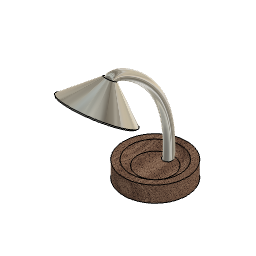
lamp-f3d (Autodesk Fusion 360 design; units mm, degrees)
Autodesk Fusion 360 part; units mm, degrees
sketch "Sketch1" plane through (0, 0, 0) normal (0, 0, 1) x (1, 0, 0)
  circle A0 centre (0, 0) radius 60
  circle A1 centre (0, 0) radius 47.5
  line L0 (-47.5, 0) -> (47.5, 0) construction
  line L1 (0, 0) -> (0, 47.5) construction
  circle A2 centre (0, 23.75) radius 8.5
  dimension "d1" = 120
  dimension "d2" = -12.5
  dimension "d3" = 17
  constraint coincident A0.centre A1.centre
  constraint coincident A1 L0.start
  constraint coincident A1 L0.end
  constraint horizontal L0
  constraint coincident A1 L1.end
  constraint perpendicular L0 L1
  constraint midpoint L1 A2.centre
  measures "d1" diameter of A0
  measures "d3" diameter of A2
extrude "Extrude1" add sketch "Sketch1" along normal blind 30 contours A0 makes body 1
extrude "Extrude2" add sketch "Sketch1" along normal blind 20 contours A1 bodies 1
fillet "Fillet1" radius 15 1 edges at (-44.2855, 17.1767, 20) on bodies 1
sketch "Sketch2" plane through (0, 0, 0) normal (1, 0, 0) x (0, 1, 0)
  spline S0 degree 5 poles (23.75, 0) (24.3992, 5.1936) (25.4927, 15.4647) (26.5181, 30.5229) (26.6466, 49.8986) (24.696, 72.9054) (20.5876, 94.6237) (14.3062, 114.9444) (5.9024, 133.7275) (-4.4608, 150.807) (-16.4659, 165.9988) (-29.5606, 179.114) (-42.9747, 189.9688) (-55.8552, 198.387) (-67.3699, 204.2128) (-76.8172, 207.3258) (-82.3694, 207.602) (-85.3632, 206.576) (-86.8422, 205.3477) (-87.4524, 204.5974) knots 0 0 0 0 0 0 0.066667 0.133333 0.2 0.266667 0.333333 0.4 0.466667 0.533333 0.6 0.666667 0.733333 0.8 0.866667 0.933333 1 1 1 1 1 1
  point P0 (23.75, 0)
  point P1 (-11.1601, 158.822)
  point P2 (-74.737, 206.2928)
  constraint coincident P0 S0.start
sweep "Sweep1" add profiles "Sketch1" path "Sketch2" along S0 section 1 contours A2 separate body makes body 2
ref_plane "WorkPlane1" through (0, -114.7133, 160.9724) normal (1, 0, 0) x (0, -0.529933, -0.84804)
sketch "Sketch4" plane through (0, -113.4772, 160.1999) normal (1, 0, 0) x (0, 1, 0)
  line L0 (18.8165, 48.9019) -> (33.2332, 39.8931)
  line L1 (18.8165, 48.9019) -> (88.8165, 48.9019) construction
  line L2 (33.2332, 39.8931) -> (51.3505, -27.7217)
  line L3 (33.2332, 39.8931) -> (103.2332, 39.8931) construction
  line L4 (36.1309, 40.6696) -> (54.2483, -26.9453)
  line L5 (54.2483, -26.9453) -> (51.3505, -27.7217)
  line L6 (36.1309, 40.6696) -> (33.2332, 39.8931)
  dimension "d21" = 75
  dimension "d22" = 70
  dimension "d24" = -3
  constraint horizontal L1
  constraint coincident L0.start L1.start
  constraint horizontal L3
  constraint coincident L0.end L2.start
  constraint perpendicular L2 L5
  constraint perpendicular L2 L6
  measures "d21" angle of L2 L3
  measures "d22" distance of L0.end L2.end
revolve "Revolve2" add sketch "Sketch4" angle 360 about axis through (0, 18.7492, 374.5497) along (0, -0.529933, -0.84804) bodies 2
